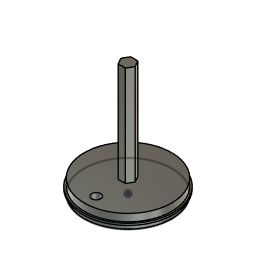
Lamp P2 (Autodesk Fusion 360 design; units mm, degrees)
Autodesk Fusion 360 part; units mm, degrees
sketch "Sketch1" plane through (0, 0, 0) normal (0, 0, 1) x (1, 0, 0)
  circle A0 centre (0, 0) radius 48
  dimension "d1" = 96
  constraint coincident A0.centre origin
  measures "d1" diameter of A0
extrude "Extrude1" add sketch "Sketch1" along normal blind 5
sketch "Sketch2" plane through (0, 0, 5) normal (0, 0, 1) x (-1, 0, 0)
  circle A0 centre (0, 0) radius 48
  circle A1 centre (0, 0) radius 50
  constraint coincident A0.centre A1.centre
extrude "Extrude2" add sketch "Sketch2" along normal blind 2 contours A0 | A1
extrude "Extrude3" add sketch "Sketch1" along normal blind 15
sketch "Sketch3" plane through (0, 0, 15) normal (0, 0, 1) x (-1, 0, 0)
  circle A0 centre (0, 0) radius 48
  line L0 (3.9499, -6.8414) -> (7.8997, 0)
  line L1 (7.8997, 0) -> (3.9499, 6.8414)
  line L2 (3.9499, 6.8414) -> (-3.9499, 6.8414)
  line L3 (-3.9499, 6.8414) -> (-7.8997, 0)
  line L4 (-7.8997, 0) -> (-3.9499, -6.8414)
  line L5 (-3.9499, -6.8414) -> (3.9499, -6.8414)
  constraint coincident A0.centre origin
extrude "Extrude4" add sketch "Sketch3" along normal blind 110 contours L0 L1 L2 L3 L4 L5
sketch "Sketch4" plane through (0, 0, 15) normal (0, 0, 1) x (-1, 0, 0)
  line L0 (-3.9499, -6.8414) -> (-7.8997, 0)
  line L1 (-7.8997, 0) -> (-3.9499, 6.8414)
  line L2 (-3.9499, 6.8414) -> (3.9499, 6.8414)
  line L3 (3.9499, 6.8414) -> (7.8997, 0)
  line L4 (7.8997, 0) -> (3.9499, -6.8414)
  line L5 (3.9499, -6.8414) -> (-3.9499, -6.8414)
  circle A0 centre (0, 0) radius 48
  circle A1 centre (0, 35) radius 5
extrude "Extrude5" cut sketch "Sketch4" against normal blind 15 contours A1
